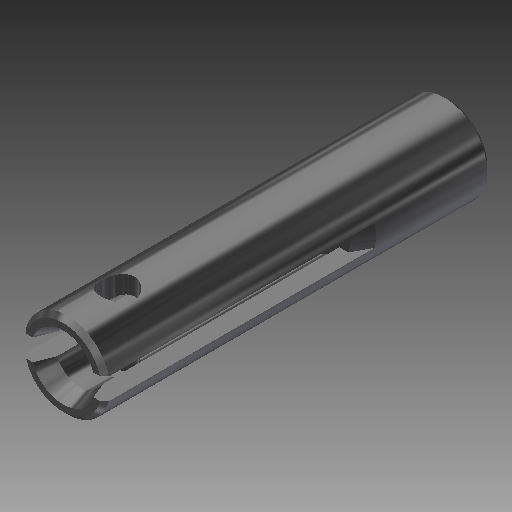
# Autodesk Inventor part: 201-02
Saved by Autodesk Inventor 2019 (Build 230136000, 136)
## iProperties
Company: Autodesk Inc.
Created: 2007-10-30
Part Number: 201-02
Document SubType Name: Modeling
Designer: Autodesk Inc.
Density: 1.425 g/cm^3
Mass: 22.9721 g
Surface Area: 90.2832 cm^2
Volume: 16.1208 cm^3
Material: Acetal Resin, Black
Description: BALL SCREW SLEEVE
Appearance: Rubber - Black - Version 1.1
Component Category: Lower Component
Author: Inventor
Autodesk Inventor part; units mm, degrees
ref_plane "YZ Plane" through (0, 0, 0) normal (1, 0, 0) x (0, 1, 0)
ref_plane "XY Plane" through (0, 0, 0) normal (0, 0, 1) x (1, 0, 0)
sketch "Sketch1" plane through (0, 0, 0) normal (0, 0, 1) x (1, 0, 0)
  circle A0 centre (0, 0) radius 10
  dimension "d0" = 20
  constraints: 1 centre point, 1 coincident
  measures "d0" diameter of A0
extrude "Extrusion1" add sketch "Sketch1" along normal mid plane 90
sketch "Sketch2" plane through (0, 0, 45) normal (0, 0, 1) x (1, 0, 0)
  circle A0 centre (0, 0) radius 6
  line L0 (-10, -2.5) -> (10, -2.5)
  line L1 (10, -2.5) -> (10, 2.5)
  line L2 (10, 2.5) -> (-10, 2.5)
  line L3 (-10, 2.5) -> (-10, -2.5)
  point P0 (-10, 0)
  point P1 (10, 0)
  dimension "d3" = 12
  dimension "d4" = 5
  dimension "d5" = 2.5
  dimension "d6" = 20
  dimension "d7" = 10
  constraints: 8 end point, 2 midpoint, 2 parallel, 1 centre point, 1 coincident, 1 horizontal, 1 perpendicular
  measures "d3" diameter of A0
  measures "d4" distance of L2.end L0.start
  measures "d5" distance from line of point (0, 0) L2
  measures "d6" distance of L1.end L2.end
  measures "d7" distance from line of point (0, 0) L3
extrude "Extrusion2" cut sketch "Sketch2" against normal blind 59
chamfer "Chamfer1" distance 1 angle 45 2 edges at (0, -10, 45) (0, 10, 45)
chamfer "Chamfer2" distance 1.5 distance2 4 1 edges at (0, 6, 45) measured on face at (-7.3096, 3.1466, 45)
chamfer "Chamfer3" distance 1.5 distance2 4 1 edges at (0, -6, 45) measured on face at (-7.3096, -3.1466, 45)
chamfer "Chamfer4" distance 4 distance2 2 1 edges at (-10, 0, -14) measured on face at (8.4358, 5.37, -15.3333)
chamfer "Chamfer5" distance 4 distance2 2 2 edges at (9.9203, 1.26, -14) (9.9203, -1.26, -14) measured on face at (8.4358, 5.37, -15.3333)
chamfer "Chamfer6" distance 1 angle 45 1 edges at (-10, 0, -45)
sketch "Sketch3" plane through (0, 0, -45) normal (0, 0, -1) x (-1, 0, 0)
  circle A0 centre (0, 0) radius 9 projected
hole "Hole1" at (0, 0, -45) direction (0, 0, 1) diameter 10.106 depth 45 thread size "M12x1.75" class "6H" standard "ANSI Metric M Profile"
sketch "Sketch4" plane through (0, 0, 0) normal (0, 1, 0) x (-1, 0, 0)
  line L0 (0, -9) -> (0, 54) projected
  circle A0 centre (0, 32.297) radius 3.95
  line L1 (-8.6458, 45) -> (8.6458, 45) projected
  point P0 (0, 0)
  dimension "d35" = 12.703
  dimension "d36" = 7.9
  constraints: 1 centre point, 1 point on line
  measures "d35" distance from line of L1 A0.centre
  measures "d36" diameter of A0
extrude "Extrusion3" cut sketch "Sketch4" along normal through all both and the other way through all
equation "\"d5\" = 0.5 * d4"
body "Solid1"
